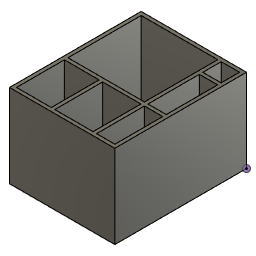
Animation v5 (Autodesk Fusion 360 archive; units mm, degrees)
design "Crate_Mid_Term"
Autodesk Fusion 360 part; units mm, degrees
note: some values were not read from the file. Set by a fixed rule: which face or edge a step refers to.
sketch "Sketch1" plane through (0, 0, 0) normal (1, 0, 0) x (0, 0, -1)
sketch "Sketch2" plane through (0, 0, 0) normal (0, 1, 0) x (1, 0, 0)
  line L0 (0, 0) -> (-24, 0)
  line L1 (-24, 0) -> (-24, -30)
  line L2 (-24, -30) -> (0, -30)
  line L3 (0, -30) -> (0, 0)
  constraint horizontal L0
  constraint vertical L1
  constraint horizontal L2
  constraint vertical L3
  constraint coincident L0.start L3.end
extrude "Extrude1" add sketch "Sketch2" along normal blind 19
sketch "Sketch3" plane through (0, 19, 0) normal (0, 1, 0) x (-1, 0, 0)
  line L0 (0, 30) -> (0, 0)
  line L1 (0, 0) -> (24, 0)
  line L2 (24, 0) -> (24, 30)
  line L3 (24, 30) -> (0, 30)
  line L4 (0.8, 0.8) -> (23.2, 0.8)
  line L5 (23.2, 0.8) -> (23.2, 29.2)
  line L6 (23.2, 29.2) -> (0.8, 29.2)
  line L7 (0.8, 29.2) -> (0.8, 0.8)
  dimension "d3" = -0.8
extrude "Extrude2" cut sketch "Sketch3" against normal blind 18.04 contours L4 L5 L6 L7
sketch "Sketch4" plane through (0, 0.96, 0) normal (0, 1, 0) x (-1, 0, 0)
  line L0 (0.8, 29.2) -> (0.8, 0.8)
  line L1 (0.8, 0.8) -> (23.2, 0.8)
  line L2 (23.2, 0.8) -> (23.2, 29.2)
  line L3 (23.2, 29.2) -> (0.8, 29.2)
  line L4 (4.9651, 0.8) -> (5.7651, 0.8)
  line L5 (5.7651, 0.8) -> (5.7651, 29.2)
  line L6 (5.7651, 29.2) -> (4.9651, 29.2)
  line L7 (4.9651, 29.2) -> (4.9651, 0.8)
  dimension "d6" = 0.8
  constraint horizontal L4
  constraint vertical L5
  constraint horizontal L6
  constraint vertical L7
  constraint coincident L3 L5.end
  constraint coincident L1 L4.start
  measures "d6" distance of L4.start L4.end
extrude "Extrude3" add sketch "Sketch4" along normal blind 18.04 contours L1 L3 L4 L5 L6 L7
sketch "Sketch5" plane through (0, 0.96, 0) normal (0, 1, 0) x (-1, 0, 0)
  line L0 (4.9651, 0.8) -> (4.9651, 29.2)
  line L1 (4.9651, 29.2) -> (0.8, 29.2)
  line L2 (0.8, 29.2) -> (0.8, 0.8)
  line L3 (0.8, 0.8) -> (4.9651, 0.8)
  line L4 (4.9651, 4.9845) -> (0.8, 4.9845)
  line L5 (0.8, 4.9845) -> (0.8, 5.7845)
  line L6 (0.8, 5.7845) -> (4.9651, 5.7845)
  line L7 (4.9651, 5.7845) -> (4.9651, 4.9845)
  dimension "d9" = 0.8
  constraint horizontal L4
  constraint vertical L5
  constraint horizontal L6
  constraint vertical L7
  constraint coincident L0 L4.start
  measures "d9" distance of L4.start L6.end
extrude "Extrude4" add sketch "Sketch5" along normal blind 18.04 contours L0 L2 L4 L5 L6 L7
sketch "Sketch6" plane through (0, 0.96, 0) normal (0, 1, 0) x (-1, 0, 0)
  line L0 (0.8, 5.7845) -> (4.9651, 5.7845)
  line L1 (4.9651, 5.7845) -> (4.9651, 29.2)
  line L2 (4.9651, 29.2) -> (0.8, 29.2)
  line L3 (0.8, 29.2) -> (0.8, 5.7845)
  line L4 (4.9651, 17.4923) -> (0.8, 17.4923)
  line L5 (0.8, 17.4923) -> (0.8, 18.2923)
  line L6 (0.8, 18.2923) -> (4.9651, 18.2923)
  line L7 (4.9651, 18.2923) -> (4.9651, 17.4923)
  dimension "d12" = 0.8
  constraint horizontal L4
  constraint vertical L5
  constraint horizontal L6
  constraint vertical L7
  constraint midpoint L1 L4.start
  measures "d12" distance of L4.start L6.end
extrude "Extrude5" add sketch "Sketch6" along normal blind 18.04 contours L1 L3 L4 L5 L6 L7
sketch "Sketch7" plane through (0, 0.96, 0) normal (0, 1, 0) x (-1, 0, 0)
  line L0 (5.7651, 29.2) -> (5.7651, 0.8)
  line L1 (5.7651, 0.8) -> (23.2, 0.8)
  line L2 (23.2, 0.8) -> (23.2, 29.2)
  line L3 (23.2, 29.2) -> (5.7651, 29.2)
  line L4 (5.7651, 17.4851) -> (23.2, 17.4851)
  line L5 (23.2, 17.4851) -> (23.2, 18.2851)
  line L6 (23.2, 18.2851) -> (5.7651, 18.2851)
  line L7 (5.7651, 18.2851) -> (5.7651, 17.4851)
  dimension "d15" = 0.8
  constraint horizontal L4
  constraint vertical L5
  constraint horizontal L6
  constraint vertical L7
  constraint coincident L0 L4.start
  measures "d15" distance of L4.start L6.end
extrude "Extrude6" add sketch "Sketch7" along normal blind 18.04 contours L0 L2 L4 L5 L6 L7
delete_face "DeleteFace1" 1 faces at (-17.3884, 6.9733, 18.2851)
sketch "Sketch8" plane through (0, 19, 0) normal (0, 1, 0) x (-1, 0, 0)
  line L0 (4.9651, 18.2923) -> (0.8, 18.2923)
  line L1 (0.8, 18.2923) -> (0.8, 29.2)
  line L2 (0.8, 29.2) -> (4.9651, 29.2)
  line L3 (4.9651, 29.2) -> (4.9651, 18.2923)
  line L4 (4.9651, 4.9845) -> (4.9651, 0.8)
  line L5 (4.9651, 0.8) -> (0.8, 0.8)
  line L6 (0.8, 0.8) -> (0.8, 4.9845)
  line L7 (0.8, 4.9845) -> (4.9651, 4.9845)
  line L8 (4.9651, 17.4923) -> (4.9651, 5.7845)
  line L9 (4.9651, 5.7845) -> (0.8, 5.7845)
  line L10 (0.8, 5.7845) -> (0.8, 17.4923)
  line L11 (0.8, 17.4923) -> (4.9651, 17.4923)
  line L12 (0, 0) -> (24, 0)
  line L13 (24, 0) -> (24, 30)
  line L14 (24, 30) -> (0, 30)
  line L15 (0, 30) -> (0, 0)
  line L16 (23.2, 17.4851) -> (23.2, 0.8)
  line L17 (23.2, 0.8) -> (5.7651, 0.8)
  line L18 (5.7651, 0.8) -> (5.7651, 17.4851)
  line L19 (5.7651, 17.4851) -> (23.2, 17.4851)
  line L20 (5.7651, 18.2923) -> (23.2, 18.2923)
  line L21 (23.2, 18.2923) -> (23.2, 29.2003)
  line L22 (23.2, 29.2003) -> (5.7651, 29.2003)
  line L23 (5.7651, 29.2003) -> (5.7651, 18.2923)
  dimension "d18" = 10.908
  constraint horizontal L20
  constraint vertical L21
  constraint horizontal L22
  constraint vertical L23
  measures "d18" distance of L20.start L22.end
extrude "Extrude7" cut sketch "Sketch8" against normal blind 18.04 contours L20 L21 L22 L23
sketch "Sketch9" plane through (0, 0.96, 0) normal (0, 1, 0) x (-1, 0, 0)
  line L0 (5.7651, 29.2003) -> (5.7651, 18.2923)
  line L1 (5.7651, 18.2923) -> (23.2, 18.2923)
  line L2 (23.2, 18.2923) -> (23.2, 29.2003)
  line L3 (23.2, 29.2003) -> (5.7651, 29.2003)
  line L4 (14.4825, 18.2923) -> (15.2825, 18.2923)
  line L5 (15.2825, 18.2923) -> (15.2825, 29.2003)
  line L6 (15.2825, 29.2003) -> (14.4825, 29.2003)
  line L7 (14.4825, 29.2003) -> (14.4825, 18.2923)
  dimension "d21" = 0.8
  constraint horizontal L4
  constraint vertical L5
  constraint horizontal L6
  constraint vertical L7
  constraint midpoint L1 L4.start
  measures "d21" distance of L4.start L4.end
extrude "Extrude8" add sketch "Sketch9" along normal blind 18.04 contours L1 L3 L4 L5 L6 L7

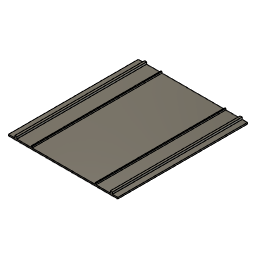
design "Floor"
Autodesk Fusion 360 part; units mm, degrees
sketch "Sketch1" plane through (0, 0, 0) normal (0, 1, 0) x (1, 0, 0)
  line L0 (0, 0) -> (-140, 0)
  line L1 (-140, 0) -> (-140, 140)
  line L2 (-140, 140) -> (0, 140)
  line L3 (0, 140) -> (0, 0)
  dimension "d1" = 140
  dimension "d2" = 140
  constraint horizontal L0
  constraint vertical L1
  constraint horizontal L2
  constraint vertical L3
  constraint coincident L0.start L3.end
  measures "d1" distance of L0.start L0.end
  measures "d2" distance of L0.start L2.end
extrude "Extrude1" add sketch "Sketch1" along normal blind 2 makes body 1
sketch "Sketch2" plane through (0, 2, 0) normal (0, 1, 0) x (-1, 0, 0)
  line L0 (0, -140) -> (140, -140)
  line L1 (140, -140) -> (140, 0)
  line L2 (140, 0) -> (0, 0)
  line L3 (0, 0) -> (0, -140)
  line L4 (70, -140) -> (23, -140)
  line L5 (117, -140) -> (116, -140)
  line L6 (117, -140) -> (117.75, -140)
  line L7 (117.75, -140) -> (116.25, -140)
  line L8 (117.75, -140) -> (116.25, -140)
  line L9 (116.25, -140) -> (116.25, 0)
  line L10 (116.25, 0) -> (117.75, 0)
  line L11 (117.75, 0) -> (117.75, -140)
  dimension "d5" = 47
  dimension "d6" = 47
  dimension "d7" = 0.75
  dimension "d8" = 1.5
  constraint midpoint L0 L4.start
  constraint parallel L0 L4
  constraint parallel L0 L6
  constraint horizontal L7
  constraint horizontal L8
  constraint vertical L9
  constraint horizontal L10
  constraint vertical L11
  constraint coincident L2 L9.end
  measures "d5" distance of L4.start L5.start
  measures "d6" distance of L4.start L4.end
  measures "d7" distance of L5.start L6.end
  measures "d8" distance of L6.end L7.end
extrude "Extrude2" add sketch "Sketch2" along normal blind 2 contours L0 L2 L5 L6 L7 L8 L9 L10 L11 bodies 1
sketch "Sketch3" plane through (0, 2, 0) normal (0, 1, 0) x (-1, 0, 0)
  line L0 (116.25, -140) -> (116.25, 0)
  line L1 (116.25, 0) -> (0, 0)
  line L2 (0, 0) -> (0, -140)
  line L3 (0, -140) -> (116.25, -140)
  line L4 (0, -140) -> (22.25, -140)
  line L5 (22.25, -140) -> (20.75, -140)
  line L6 (20.75, -140) -> (20.75, 0)
  line L7 (20.75, 0) -> (22.25, 0)
  line L8 (22.25, 0) -> (22.25, -140)
  dimension "d11" = 22.25
  dimension "d12" = 1.5
  constraint coincident L2.end L3.start
  constraint perpendicular L2 L4
  constraint horizontal L5
  constraint vertical L6
  constraint horizontal L7
  constraint vertical L8
  measures "d11" distance of L2.end L4.end
  measures "d12" distance of L4.end L5.end
extrude "Extrude3" add sketch "Sketch3" along normal blind 2 contours L1 L3 L4 L5 L6 L7 L8 bodies 1
sketch "Sketch4" plane through (0, 2, 0) normal (0, 1, 0) x (-1, 0, 0)
extrude "Extrude4" add 1 faces at (0, 0.6667, -93.3333) along direction (1, 0, 0) blind 10 on bodies 1 bodies 1
extrude "Extrude5" add 1 faces at (-140, 0.6667, -46.6667) along direction (-1, 0, 0) blind 10 on bodies 1 bodies 1
sketch "Sketch5" plane through (0, 2, 0) normal (0, 1, 0) x (-1, 0, 0)
  line L0 (20.75, -140) -> (20.75, 0)
  line L1 (20.75, 0) -> (-10, 0)
  line L2 (-10, 0) -> (-10, -140)
  line L3 (-10, -140) -> (20.75, -140)
  line L4 (0.75, -140) -> (-2.25, -140)
  line L5 (-2.25, -140) -> (-2.25, 0)
  line L6 (-2.25, 0) -> (0.75, 0)
  line L7 (0.75, 0) -> (0.75, -140)
  dimension "d19" = 20
  dimension "d20" = 3
  dimension "d21" = 140
  constraint horizontal L4
  constraint vertical L5
  constraint horizontal L6
  constraint vertical L7
  measures "d19" distance of L0.start L4.start
  measures "d20" distance of L4.start L4.end
  measures "d21" distance of L4.start L6.end
extrude "Extrude6" add sketch "Sketch5" along normal blind 3 contours L1 L3 L4 L5 L6 L7 bodies 1
sketch "Sketch6" plane through (0, 2, 0) normal (0, 1, 0) x (-1, 0, 0)
  line L0 (117.75, 0) -> (117.75, -140)
  line L1 (117.75, -140) -> (150, -140)
  line L2 (150, -140) -> (150, 0)
  line L3 (150, 0) -> (117.75, 0)
  line L4 (137.75, -140) -> (140.75, -140)
  line L5 (140.75, -140) -> (140.75, 0)
  line L6 (140.75, 0) -> (137.75, 0)
  line L7 (137.75, 0) -> (137.75, -140)
  dimension "d24" = 20
  dimension "d25" = 3
  dimension "d26" = 140
  constraint horizontal L4
  constraint vertical L5
  constraint horizontal L6
  constraint vertical L7
  measures "d24" distance of L0.end L4.start
  measures "d25" distance of L4.start L4.end
  measures "d26" distance of L4.start L6.end
extrude "Extrude7" add sketch "Sketch6" along normal blind 3 contours L1 L3 L4 L5 L6 L7 bodies 1
sketch "Sketch7" plane through (0, 5, 0) normal (0, 1, 0) x (-1, 0, 0)
sketch "Sketch8" plane through (0, 2, 0) normal (0, 1, 0) x (-1, 0, 0)
sketch "Sketch9" plane through (0, 5, 0) normal (0, 1, 0) x (-1, 0, 0)
sketch "Sketch10" plane through (0, 5, 0) normal (0, 1, 0) x (-1, 0, 0)
sketch "Sketch11" plane through (0, 2, 0) normal (0, 1, 0) x (-1, 0, 0)
  line L0 (22.25, -140) -> (116.25, -140)
  line L1 (116.25, -140) -> (116.25, 0)
  line L2 (116.25, 0) -> (22.25, 0)
  line L3 (23.25, 0) -> (21.75, 0)
  line L4 (21.75, 0) -> (21.75, -140)
  line L5 (21.75, -140) -> (23.25, -140)
  line L6 (23.25, -140) -> (23.25, 0)
  dimension "d29" = 1
  dimension "d30" = 1.5
  constraint horizontal L3
  constraint vertical L4
  constraint horizontal L5
  constraint vertical L6
  measures "d29" distance of L2.end L3.start
  measures "d30" distance of L3.start L3.end
extrude "Extrude8" cut 1 faces at (-21.75, 4, -93.3333) along direction (0, -1, 0) blind 2 on bodies 1 bodies 1
extrude "Extrude9" add sketch "Sketch11" along normal blind 2 contours L0 L2 L3 L4 L5 L6 bodies 1
extrude "Extrude10" cut 1 faces at (-116.75, 4, -93.3333) along direction (0, -1, 0) blind 2 on bodies 1 bodies 1
sketch "Sketch12" plane through (0, 2, 0) normal (0, 1, 0) x (-1, 0, 0)
  line L0 (23.25, 0) -> (23.25, -140)
  line L1 (23.25, -140) -> (137.75, -140)
  line L2 (137.75, -140) -> (137.75, 0)
  line L3 (137.75, 0) -> (23.25, 0)
  line L4 (23.25, -140) -> (115.25, -140)
  line L5 (115.25, -140) -> (116.75, -140)
  line L6 (116.75, -140) -> (116.75, 0)
  line L7 (116.75, 0) -> (115.25, 0)
  line L8 (115.25, 0) -> (115.25, -140)
  dimension "d37" = 92
  dimension "d38" = 1.5
  constraint coincident L0.end L1.start
  constraint perpendicular L0 L4
  constraint horizontal L5
  constraint vertical L6
  constraint horizontal L7
  constraint vertical L8
  measures "d37" distance of L0.end L4.end
  measures "d38" distance of L4.end L5.end
extrude "Extrude11" add sketch "Sketch12" along normal blind 2 contours L1 L3 L5 L6 L7 L8 bodies 1
sketch "Sketch13" plane through (0, 2, 0) normal (0, 1, 0) x (-1, 0, 0)
copy_body "Body->Comp1" bodies 1 removing the originals makes body 2 in component "Component"
extrude "Extrude1'" add 1 faces at (-92.5833, 0.6667, 0) along direction (0, 0, 1) blind 50 on bodies 2 bodies 2 in component "Component"
component "Component" placed x (1, 0, 0) y (0, 1, 0) z (0, 0, 1) at (0, 0, 0)

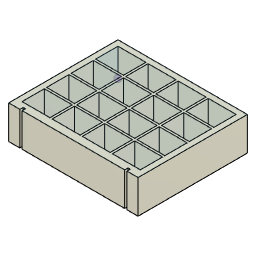
design "Cabinet"
Autodesk Fusion 360 part; units mm, degrees
sketch "Sketch1" plane through (0, 0, 0) normal (0, 1, 0) x (1, 0, 0)
sketch "Sketch2" plane through (0, 0, 0) normal (0, 1, 0) x (1, 0, 0)
sketch "Sketch3" plane through (0, 0, 0) normal (0, 1, 0) x (1, 0, 0)
  line L0 (-10, 10) -> (100, 10)
  line L1 (100, 10) -> (100, -80)
  line L2 (100, -80) -> (-10, -80)
  line L3 (-10, -80) -> (-10, 10)
  constraint horizontal L0
  constraint vertical L1
  constraint horizontal L2
  constraint vertical L3
sketch "Sketch4" plane through (0, 0, 0) normal (0, 1, 0) x (1, 0, 0)
sketch "Sketch5" plane through (0, 0, 0) normal (0, 1, 0) x (1, 0, 0)
  line L0 (0, 0) -> (116, 0)
  line L1 (116, 0) -> (116, -98)
  line L2 (116, -98) -> (0, -98)
  line L3 (0, -98) -> (0, 0)
  dimension "d4" = 116
  dimension "d5" = 98
  constraint horizontal L0
  constraint vertical L1
  constraint horizontal L2
  constraint vertical L3
  constraint coincident L0.start L3.end
  measures "d4" distance of L0.start L0.end
  measures "d5" distance of L0.start L2.end
extrude "Extrude2" add sketch "Sketch5" along normal blind 30
shell "Shell2" thickness 5 removed faces 1 at (38.6667, 30, 32.6667)
delete_face "DeleteFace2" 1 faces at (40.3333, 5, 34.3333)
sketch "Sketch6" plane through (0, 0, 0) normal (0, 1, 0) x (1, 0, 0)
  line L0 (5, -5) -> (32, -5)
  line L1 (32, -5) -> (32, -27)
  line L2 (32, -27) -> (5, -27)
  line L3 (5, -27) -> (5, -5)
  dimension "d9" = 27
  dimension "d10" = 22
  constraint horizontal L0
  constraint vertical L1
  constraint horizontal L2
  constraint vertical L3
  measures "d9" distance of L0.start L0.end
  measures "d10" distance of L0.start L2.end
extrude "Extrude3" add sketch "Sketch6" along normal blind 30
sketch "Sketch7" plane through (0, 30, 0) normal (0, 1, 0) x (-1, 0, 0)
  line L0 (-116, 98) -> (-116, 0)
  line L1 (-116, 0) -> (0, 0)
  line L2 (0, 0) -> (0, 98)
  line L3 (0, 98) -> (-116, 98)
  line L4 (-111, 93) -> (-5, 93)
  line L5 (-5, 93) -> (-5, 27)
  line L6 (-5, 27) -> (-32, 27)
  line L7 (-32, 27) -> (-32, 5)
  line L8 (-32, 5) -> (-111, 5)
  line L9 (-111, 5) -> (-111, 93)
  line L10 (-5, 5) -> (-30, 5)
  line L11 (-30, 5) -> (-30, 25)
  line L12 (-30, 25) -> (-5, 25)
  line L13 (-5, 25) -> (-5, 5)
  constraint horizontal L10
  constraint vertical L11
  constraint horizontal L12
  constraint vertical L13
extrude "Extrude4" cut sketch "Sketch7" against normal blind 30 contours L10 L11 L12 L13
sketch "Sketch8" plane through (0, 0, 0) normal (0, 1, 0) x (1, 0, 0)
  line L0 (32, -5) -> (59, -5)
  line L1 (59, -5) -> (59, -27)
  line L2 (59, -27) -> (32, -27)
  line L3 (32, -27) -> (32, -5)
  dimension "d15" = 27
  dimension "d16" = 22
  constraint horizontal L0
  constraint vertical L1
  constraint horizontal L2
  constraint vertical L3
  measures "d15" distance of L0.start L0.end
  measures "d16" distance of L0.start L2.end
extrude "Extrude5" add sketch "Sketch8" along normal blind 30
sketch "Sketch9" plane through (0, 30, 0) normal (0, 1, 0) x (-1, 0, 0)
  line L0 (-30, 5) -> (-30, 25)
  line L1 (-30, 25) -> (-5, 25)
  line L2 (-5, 25) -> (-5, 5)
  line L3 (-5, 5) -> (-30, 5)
  line L4 (-116, 98) -> (-116, 0)
  line L5 (-116, 0) -> (0, 0)
  line L6 (0, 0) -> (0, 98)
  line L7 (0, 98) -> (-116, 98)
  line L8 (-111, 93) -> (-5, 93)
  line L9 (-5, 93) -> (-5, 27)
  line L10 (-5, 27) -> (-59, 27)
  line L11 (-59, 27) -> (-59, 5)
  line L12 (-59, 5) -> (-111, 5)
  line L13 (-111, 5) -> (-111, 93)
  line L14 (-32, 5) -> (-57, 5)
  line L15 (-57, 5) -> (-57, 25)
  line L16 (-57, 25) -> (-32, 25)
  line L17 (-32, 25) -> (-32, 5)
  constraint horizontal L14
  constraint vertical L15
  constraint horizontal L16
  constraint vertical L17
extrude "Extrude6" cut sketch "Sketch9" against normal blind 30 contours L14 L15 L16 L17
sketch "Sketch10" plane through (0, 0, 0) normal (0, 1, 0) x (1, 0, 0)
  line L0 (59, -5) -> (86, -5)
  line L1 (86, -5) -> (86, -27)
  line L2 (86, -27) -> (59, -27)
  line L3 (59, -27) -> (59, -5)
  dimension "d21" = 27
  dimension "d22" = 22
  constraint horizontal L0
  constraint vertical L1
  constraint horizontal L2
  constraint vertical L3
  measures "d21" distance of L0.start L0.end
  measures "d22" distance of L0.start L2.end
extrude "Extrude7" add sketch "Sketch10" along normal blind 30
sketch "Sketch11" plane through (0, 30, 0) normal (0, 1, 0) x (-1, 0, 0)
  line L0 (-57, 5) -> (-57, 25)
  line L1 (-57, 25) -> (-32, 25)
  line L2 (-32, 25) -> (-32, 5)
  line L3 (-32, 5) -> (-57, 5)
  line L4 (-30, 5) -> (-30, 25)
  line L5 (-30, 25) -> (-5, 25)
  line L6 (-5, 25) -> (-5, 5)
  line L7 (-5, 5) -> (-30, 5)
  line L8 (-116, 98) -> (-116, 0)
  line L9 (-116, 0) -> (0, 0)
  line L10 (0, 0) -> (0, 98)
  line L11 (0, 98) -> (-116, 98)
  line L12 (-111, 93) -> (-5, 93)
  line L13 (-5, 93) -> (-5, 27)
  line L14 (-5, 27) -> (-86, 27)
  line L15 (-86, 27) -> (-86, 5)
  line L16 (-86, 5) -> (-111, 5)
  line L17 (-111, 5) -> (-111, 93)
  line L18 (-59, 5) -> (-84, 5)
  line L19 (-84, 5) -> (-84, 25)
  line L20 (-84, 25) -> (-59, 25)
  line L21 (-59, 25) -> (-59, 5)
  constraint horizontal L18
  constraint vertical L19
  constraint horizontal L20
  constraint vertical L21
extrude "Extrude8" cut sketch "Sketch11" against normal blind 30 contours L18 L19 L20 L21
sketch "Sketch12" plane through (0, 0, 0) normal (0, 1, 0) x (1, 0, 0)
  line L0 (86, -27) -> (111, -27)
  line L1 (111, -27) -> (111, -5)
  line L2 (111, -5) -> (86, -5)
  line L3 (86, -5) -> (86, -27)
  constraint horizontal L0
  constraint vertical L1
  constraint horizontal L2
  constraint vertical L3
extrude "Extrude9" add sketch "Sketch12" along normal blind 30
sketch "Sketch13" plane through (0, 30, 0) normal (0, 1, 0) x (-1, 0, 0)
  line L0 (-84, 5) -> (-84, 25)
  line L1 (-84, 25) -> (-59, 25)
  line L2 (-59, 25) -> (-59, 5)
  line L3 (-59, 5) -> (-84, 5)
  line L4 (-57, 5) -> (-57, 25)
  line L5 (-57, 25) -> (-32, 25)
  line L6 (-32, 25) -> (-32, 5)
  line L7 (-32, 5) -> (-57, 5)
  line L8 (-30, 5) -> (-30, 25)
  line L9 (-30, 25) -> (-5, 25)
  line L10 (-5, 25) -> (-5, 5)
  line L11 (-5, 5) -> (-30, 5)
  line L12 (-116, 98) -> (-116, 0)
  line L13 (-116, 0) -> (0, 0)
  line L14 (0, 0) -> (0, 98)
  line L15 (0, 98) -> (-116, 98)
  line L16 (-111, 93) -> (-5, 93)
  line L17 (-5, 93) -> (-5, 27)
  line L18 (-5, 27) -> (-111, 27)
  line L19 (-111, 27) -> (-111, 93)
  line L20 (-86, 25) -> (-111, 25)
  line L21 (-111, 25) -> (-111, 5)
  line L22 (-111, 5) -> (-86, 5)
  line L23 (-86, 5) -> (-86, 25)
  constraint horizontal L20
  constraint vertical L21
  constraint horizontal L22
  constraint vertical L23
extrude "Extrude10" cut sketch "Sketch13" against normal blind 30 contours L20 L21 L22 L23
sketch "Sketch14" plane through (0, 0, 0) normal (0, 1, 0) x (1, 0, 0)
  line L0 (5, -27) -> (32, -27)
  line L1 (32, -27) -> (32, -49)
  line L2 (32, -49) -> (5, -49)
  line L3 (5, -49) -> (5, -27)
  constraint horizontal L0
  constraint vertical L1
  constraint horizontal L2
  constraint vertical L3
extrude "Extrude11" add sketch "Sketch14" along normal blind 30
sketch "Sketch15" plane through (0, 30, 0) normal (0, 1, 0) x (-1, 0, 0)
  line L0 (-111, 25) -> (-86, 25)
  line L1 (-86, 25) -> (-86, 5)
  line L2 (-86, 5) -> (-111, 5)
  line L3 (-111, 5) -> (-111, 25)
  line L4 (-84, 5) -> (-84, 25)
  line L5 (-84, 25) -> (-59, 25)
  line L6 (-59, 25) -> (-59, 5)
  line L7 (-59, 5) -> (-84, 5)
  line L8 (-57, 5) -> (-57, 25)
  line L9 (-57, 25) -> (-32, 25)
  line L10 (-32, 25) -> (-32, 5)
  line L11 (-32, 5) -> (-57, 5)
  line L12 (-30, 5) -> (-30, 25)
  line L13 (-30, 25) -> (-5, 25)
  line L14 (-5, 25) -> (-5, 5)
  line L15 (-5, 5) -> (-30, 5)
  line L16 (-116, 98) -> (-116, 0)
  line L17 (-116, 0) -> (0, 0)
  line L18 (0, 0) -> (0, 98)
  line L19 (0, 98) -> (-116, 98)
  line L20 (-111, 93) -> (-5, 93)
  line L21 (-5, 93) -> (-5, 49)
  line L22 (-5, 49) -> (-32, 49)
  line L23 (-32, 49) -> (-32, 27)
  line L24 (-32, 27) -> (-111, 27)
  line L25 (-111, 27) -> (-111, 93)
  line L26 (-5, 27) -> (-30, 27)
  line L27 (-30, 27) -> (-30, 47)
  line L28 (-30, 47) -> (-5, 47)
  line L29 (-5, 47) -> (-5, 27)
  constraint horizontal L26
  constraint vertical L27
  constraint horizontal L28
  constraint vertical L29
extrude "Extrude12" cut sketch "Sketch15" against normal blind 30 contours L26 L27 L28 L29
sketch "Sketch16" plane through (5, 0, 0) normal (1, 0, 0) x (0, 0, -1)
  line L0 (-5, 30) -> (-25, 30)
  line L1 (-25, 30) -> (-25, 0)
  line L2 (-25, 0) -> (-5, 0)
  line L3 (-5, 0) -> (-5, 30)
sketch "Sketch17" plane through (0, 0, 0) normal (0, 1, 0) x (1, 0, 0)
  line L0 (32, -49) -> (59, -49)
  line L1 (59, -49) -> (59, -27)
  line L2 (59, -27) -> (32, -27)
  line L3 (32, -27) -> (32, -49)
  constraint horizontal L0
  constraint vertical L1
  constraint horizontal L2
  constraint vertical L3
extrude "Extrude13" add sketch "Sketch17" along normal blind 30
sketch "Sketch18" plane through (0, 30, 0) normal (0, 1, 0) x (-1, 0, 0)
  line L0 (-30, 27) -> (-30, 47)
  line L1 (-30, 47) -> (-5, 47)
  line L2 (-5, 47) -> (-5, 27)
  line L3 (-5, 27) -> (-30, 27)
  line L4 (-111, 25) -> (-86, 25)
  line L5 (-86, 25) -> (-86, 5)
  line L6 (-86, 5) -> (-111, 5)
  line L7 (-111, 5) -> (-111, 25)
  line L8 (-84, 5) -> (-84, 25)
  line L9 (-84, 25) -> (-59, 25)
  line L10 (-59, 25) -> (-59, 5)
  line L11 (-59, 5) -> (-84, 5)
  line L12 (-57, 5) -> (-57, 25)
  line L13 (-57, 25) -> (-32, 25)
  line L14 (-32, 25) -> (-32, 5)
  line L15 (-32, 5) -> (-57, 5)
  line L16 (-30, 5) -> (-30, 25)
  line L17 (-30, 25) -> (-5, 25)
  line L18 (-5, 25) -> (-5, 5)
  line L19 (-5, 5) -> (-30, 5)
  line L20 (-116, 98) -> (-116, 0)
  line L21 (-116, 0) -> (0, 0)
  line L22 (0, 0) -> (0, 98)
  line L23 (0, 98) -> (-116, 98)
  line L24 (-111, 93) -> (-5, 93)
  line L25 (-5, 93) -> (-5, 49)
  line L26 (-5, 49) -> (-59, 49)
  line L27 (-59, 49) -> (-59, 27)
  line L28 (-59, 27) -> (-111, 27)
  line L29 (-111, 27) -> (-111, 93)
  line L30 (-32, 27) -> (-57, 27)
  line L31 (-57, 27) -> (-57, 47)
  line L32 (-57, 47) -> (-32, 47)
  line L33 (-32, 47) -> (-32, 27)
  constraint horizontal L30
  constraint vertical L31
  constraint horizontal L32
  constraint vertical L33
extrude "Extrude14" cut sketch "Sketch18" against normal blind 30 contours L30 L31 L32 L33
sketch "Sketch19" plane through (0, 0, 0) normal (0, 1, 0) x (1, 0, 0)
  line L0 (59, -49) -> (86, -49)
  line L1 (86, -49) -> (86, -27)
  line L2 (86, -27) -> (59, -27)
  line L3 (59, -27) -> (59, -49)
  constraint horizontal L0
  constraint vertical L1
  constraint horizontal L2
  constraint vertical L3
extrude "Extrude15" add sketch "Sketch19" along normal blind 30
sketch "Sketch20" plane through (0, 0, 0) normal (0, 1, 0) x (1, 0, 0)
  line L0 (86, -27) -> (111, -27)
  line L1 (111, -27) -> (111, -49)
  line L2 (111, -49) -> (86, -49)
  line L3 (86, -49) -> (86, -27)
  constraint horizontal L0
  constraint vertical L1
  constraint horizontal L2
  constraint vertical L3
extrude "Extrude16" add sketch "Sketch20" along normal blind 30
sketch "Sketch21" plane through (0, 30, 0) normal (0, 1, 0) x (-1, 0, 0)
  line L0 (-57, 27) -> (-57, 47)
  line L1 (-57, 47) -> (-32, 47)
  line L2 (-32, 47) -> (-32, 27)
  line L3 (-32, 27) -> (-57, 27)
  line L4 (-30, 27) -> (-30, 47)
  line L5 (-30, 47) -> (-5, 47)
  line L6 (-5, 47) -> (-5, 27)
  line L7 (-5, 27) -> (-30, 27)
  line L8 (-111, 25) -> (-86, 25)
  line L9 (-86, 25) -> (-86, 5)
  line L10 (-86, 5) -> (-111, 5)
  line L11 (-111, 5) -> (-111, 25)
  line L12 (-84, 5) -> (-84, 25)
  line L13 (-84, 25) -> (-59, 25)
  line L14 (-59, 25) -> (-59, 5)
  line L15 (-59, 5) -> (-84, 5)
  line L16 (-57, 5) -> (-57, 25)
  line L17 (-57, 25) -> (-32, 25)
  line L18 (-32, 25) -> (-32, 5)
  line L19 (-32, 5) -> (-57, 5)
  line L20 (-30, 5) -> (-30, 25)
  line L21 (-30, 25) -> (-5, 25)
  line L22 (-5, 25) -> (-5, 5)
  line L23 (-5, 5) -> (-30, 5)
  line L24 (-116, 98) -> (-116, 0)
  line L25 (-116, 0) -> (0, 0)
  line L26 (0, 0) -> (0, 98)
  line L27 (0, 98) -> (-116, 98)
  line L28 (-111, 93) -> (-5, 93)
  line L29 (-5, 93) -> (-5, 49)
  line L30 (-5, 49) -> (-111, 49)
  line L31 (-111, 49) -> (-111, 93)
  line L32 (-59, 27) -> (-84, 27)
  line L33 (-84, 27) -> (-84, 47)
  line L34 (-84, 47) -> (-59, 47)
  line L35 (-59, 47) -> (-59, 27)
  constraint horizontal L32
  constraint vertical L33
  constraint horizontal L34
  constraint vertical L35
extrude "Extrude17" cut sketch "Sketch21" against normal blind 30 contours L32 L33 L34 L35
sketch "Sketch22" plane through (0, 30, 0) normal (0, 1, 0) x (-1, 0, 0)
  line L0 (-84, 27) -> (-84, 47)
  line L1 (-84, 47) -> (-59, 47)
  line L2 (-59, 47) -> (-59, 27)
  line L3 (-59, 27) -> (-84, 27)
  line L4 (-57, 27) -> (-57, 47)
  line L5 (-57, 47) -> (-32, 47)
  line L6 (-32, 47) -> (-32, 27)
  line L7 (-32, 27) -> (-57, 27)
  line L8 (-30, 27) -> (-30, 47)
  line L9 (-30, 47) -> (-5, 47)
  line L10 (-5, 47) -> (-5, 27)
  line L11 (-5, 27) -> (-30, 27)
  line L12 (-111, 25) -> (-86, 25)
  line L13 (-86, 25) -> (-86, 5)
  line L14 (-86, 5) -> (-111, 5)
  line L15 (-111, 5) -> (-111, 25)
  line L16 (-84, 5) -> (-84, 25)
  line L17 (-84, 25) -> (-59, 25)
  line L18 (-59, 25) -> (-59, 5)
  line L19 (-59, 5) -> (-84, 5)
  line L20 (-57, 5) -> (-57, 25)
  line L21 (-57, 25) -> (-32, 25)
  line L22 (-32, 25) -> (-32, 5)
  line L23 (-32, 5) -> (-57, 5)
  line L24 (-30, 5) -> (-30, 25)
  line L25 (-30, 25) -> (-5, 25)
  line L26 (-5, 25) -> (-5, 5)
  line L27 (-5, 5) -> (-30, 5)
  line L28 (-116, 98) -> (-116, 0)
  line L29 (-116, 0) -> (0, 0)
  line L30 (0, 0) -> (0, 98)
  line L31 (0, 98) -> (-116, 98)
  line L32 (-111, 93) -> (-5, 93)
  line L33 (-5, 93) -> (-5, 49)
  line L34 (-5, 49) -> (-111, 49)
  line L35 (-111, 49) -> (-111, 93)
  line L36 (-86, 27) -> (-111, 27)
  line L37 (-111, 27) -> (-111, 47)
  line L38 (-111, 47) -> (-86, 47)
  line L39 (-86, 47) -> (-86, 27)
  constraint horizontal L36
  constraint vertical L37
  constraint horizontal L38
  constraint vertical L39
extrude "Extrude18" cut sketch "Sketch22" against normal blind 30 contours L36 L37 L38 L39
sketch "Sketch23" plane through (0, 0, 0) normal (0, 1, 0) x (1, 0, 0)
  line L0 (5, -49) -> (111, -49)
  line L1 (111, -49) -> (111, -93)
  line L2 (111, -93) -> (5, -93)
  line L3 (5, -93) -> (5, -49)
  constraint horizontal L0
  constraint vertical L1
  constraint horizontal L2
  constraint vertical L3
extrude "Extrude19" add sketch "Sketch23" along normal blind 30
sketch "Sketch24" plane through (0, 30, 0) normal (0, 1, 0) x (-1, 0, 0)
  line L0 (-111, 27) -> (-111, 47)
  line L1 (-111, 47) -> (-86, 47)
  line L2 (-86, 47) -> (-86, 27)
  line L3 (-86, 27) -> (-111, 27)
  line L4 (-84, 27) -> (-84, 47)
  line L5 (-84, 47) -> (-59, 47)
  line L6 (-59, 47) -> (-59, 27)
  line L7 (-59, 27) -> (-84, 27)
  line L8 (-57, 27) -> (-57, 47)
  line L9 (-57, 47) -> (-32, 47)
  line L10 (-32, 47) -> (-32, 27)
  line L11 (-32, 27) -> (-57, 27)
  line L12 (-30, 27) -> (-30, 47)
  line L13 (-30, 47) -> (-5, 47)
  line L14 (-5, 47) -> (-5, 27)
  line L15 (-5, 27) -> (-30, 27)
  line L16 (-111, 25) -> (-86, 25)
  line L17 (-86, 25) -> (-86, 5)
  line L18 (-86, 5) -> (-111, 5)
  line L19 (-111, 5) -> (-111, 25)
  line L20 (-84, 5) -> (-84, 25)
  line L21 (-84, 25) -> (-59, 25)
  line L22 (-59, 25) -> (-59, 5)
  line L23 (-59, 5) -> (-84, 5)
  line L24 (-57, 5) -> (-57, 25)
  line L25 (-57, 25) -> (-32, 25)
  line L26 (-32, 25) -> (-32, 5)
  line L27 (-32, 5) -> (-57, 5)
  line L28 (-30, 5) -> (-30, 25)
  line L29 (-30, 25) -> (-5, 25)
  line L30 (-5, 25) -> (-5, 5)
  line L31 (-5, 5) -> (-30, 5)
  line L32 (-116, 98) -> (-116, 0)
  line L33 (-116, 0) -> (0, 0)
  line L34 (0, 0) -> (0, 98)
  line L35 (0, 98) -> (-116, 98)
  line L36 (-5, 49) -> (-30, 49)
  line L37 (-30, 49) -> (-30, 69)
  line L38 (-30, 69) -> (-5, 69)
  line L39 (-5, 69) -> (-5, 49)
  constraint horizontal L36
  constraint vertical L37
  constraint horizontal L38
  constraint vertical L39
extrude "Extrude20" cut sketch "Sketch24" against normal blind 30 contours L36 L37 L38 L39
sketch "Sketch25" plane through (0, 30, 0) normal (0, 1, 0) x (-1, 0, 0)
  line L0 (-30, 49) -> (-30, 69)
  line L1 (-30, 69) -> (-5, 69)
  line L2 (-5, 69) -> (-5, 49)
  line L3 (-5, 49) -> (-30, 49)
  line L4 (-111, 27) -> (-111, 47)
  line L5 (-111, 47) -> (-86, 47)
  line L6 (-86, 47) -> (-86, 27)
  line L7 (-86, 27) -> (-111, 27)
  line L8 (-84, 27) -> (-84, 47)
  line L9 (-84, 47) -> (-59, 47)
  line L10 (-59, 47) -> (-59, 27)
  line L11 (-59, 27) -> (-84, 27)
  line L12 (-57, 27) -> (-57, 47)
  line L13 (-57, 47) -> (-32, 47)
  line L14 (-32, 47) -> (-32, 27)
  line L15 (-32, 27) -> (-57, 27)
  line L16 (-30, 27) -> (-30, 47)
  line L17 (-30, 47) -> (-5, 47)
  line L18 (-5, 47) -> (-5, 27)
  line L19 (-5, 27) -> (-30, 27)
  line L20 (-111, 25) -> (-86, 25)
  line L21 (-86, 25) -> (-86, 5)
  line L22 (-86, 5) -> (-111, 5)
  line L23 (-111, 5) -> (-111, 25)
  line L24 (-84, 5) -> (-84, 25)
  line L25 (-84, 25) -> (-59, 25)
  line L26 (-59, 25) -> (-59, 5)
  line L27 (-59, 5) -> (-84, 5)
  line L28 (-57, 5) -> (-57, 25)
  line L29 (-57, 25) -> (-32, 25)
  line L30 (-32, 25) -> (-32, 5)
  line L31 (-32, 5) -> (-57, 5)
  line L32 (-30, 5) -> (-30, 25)
  line L33 (-30, 25) -> (-5, 25)
  line L34 (-5, 25) -> (-5, 5)
  line L35 (-5, 5) -> (-30, 5)
  line L36 (-116, 98) -> (-116, 0)
  line L37 (-116, 0) -> (0, 0)
  line L38 (0, 0) -> (0, 98)
  line L39 (0, 98) -> (-116, 98)
  line L40 (-32, 49) -> (-57, 49)
  line L41 (-57, 49) -> (-57, 69)
  line L42 (-57, 69) -> (-32, 69)
  line L43 (-32, 69) -> (-32, 49)
  constraint horizontal L40
  constraint vertical L41
  constraint horizontal L42
  constraint vertical L43
extrude "Extrude21" cut sketch "Sketch25" against normal blind 30 contours L40 L41 L42 L43
sketch "Sketch26" plane through (0, 30, 0) normal (0, 1, 0) x (-1, 0, 0)
  line L0 (-57, 49) -> (-57, 69)
  line L1 (-57, 69) -> (-32, 69)
  line L2 (-32, 69) -> (-32, 49)
  line L3 (-32, 49) -> (-57, 49)
  line L4 (-30, 49) -> (-30, 69)
  line L5 (-30, 69) -> (-5, 69)
  line L6 (-5, 69) -> (-5, 49)
  line L7 (-5, 49) -> (-30, 49)
  line L8 (-111, 27) -> (-111, 47)
  line L9 (-111, 47) -> (-86, 47)
  line L10 (-86, 47) -> (-86, 27)
  line L11 (-86, 27) -> (-111, 27)
  line L12 (-84, 27) -> (-84, 47)
  line L13 (-84, 47) -> (-59, 47)
  line L14 (-59, 47) -> (-59, 27)
  line L15 (-59, 27) -> (-84, 27)
  line L16 (-57, 27) -> (-57, 47)
  line L17 (-57, 47) -> (-32, 47)
  line L18 (-32, 47) -> (-32, 27)
  line L19 (-32, 27) -> (-57, 27)
  line L20 (-30, 27) -> (-30, 47)
  line L21 (-30, 47) -> (-5, 47)
  line L22 (-5, 47) -> (-5, 27)
  line L23 (-5, 27) -> (-30, 27)
  line L24 (-111, 25) -> (-86, 25)
  line L25 (-86, 25) -> (-86, 5)
  line L26 (-86, 5) -> (-111, 5)
  line L27 (-111, 5) -> (-111, 25)
  line L28 (-84, 5) -> (-84, 25)
  line L29 (-84, 25) -> (-59, 25)
  line L30 (-59, 25) -> (-59, 5)
  line L31 (-59, 5) -> (-84, 5)
  line L32 (-57, 5) -> (-57, 25)
  line L33 (-57, 25) -> (-32, 25)
  line L34 (-32, 25) -> (-32, 5)
  line L35 (-32, 5) -> (-57, 5)
  line L36 (-30, 5) -> (-30, 25)
  line L37 (-30, 25) -> (-5, 25)
  line L38 (-5, 25) -> (-5, 5)
  line L39 (-5, 5) -> (-30, 5)
  line L40 (-116, 98) -> (-116, 0)
  line L41 (-116, 0) -> (0, 0)
  line L42 (0, 0) -> (0, 98)
  line L43 (0, 98) -> (-116, 98)
  line L44 (-59, 49) -> (-84, 49)
  line L45 (-84, 49) -> (-84, 69)
  line L46 (-84, 69) -> (-59, 69)
  line L47 (-59, 69) -> (-59, 49)
  constraint horizontal L44
  constraint vertical L45
  constraint horizontal L46
  constraint vertical L47
extrude "Extrude22" cut sketch "Sketch26" against normal blind 30 contours L44 L45 L46 L47
sketch "Sketch27" plane through (0, 30, 0) normal (0, 1, 0) x (-1, 0, 0)
  line L0 (-84, 49) -> (-84, 69)
  line L1 (-84, 69) -> (-59, 69)
  line L2 (-59, 69) -> (-59, 49)
  line L3 (-59, 49) -> (-84, 49)
  line L4 (-57, 49) -> (-57, 69)
  line L5 (-57, 69) -> (-32, 69)
  line L6 (-32, 69) -> (-32, 49)
  line L7 (-32, 49) -> (-57, 49)
  line L8 (-30, 49) -> (-30, 69)
  line L9 (-30, 69) -> (-5, 69)
  line L10 (-5, 69) -> (-5, 49)
  line L11 (-5, 49) -> (-30, 49)
  line L12 (-111, 27) -> (-111, 47)
  line L13 (-111, 47) -> (-86, 47)
  line L14 (-86, 47) -> (-86, 27)
  line L15 (-86, 27) -> (-111, 27)
  line L16 (-84, 27) -> (-84, 47)
  line L17 (-84, 47) -> (-59, 47)
  line L18 (-59, 47) -> (-59, 27)
  line L19 (-59, 27) -> (-84, 27)
  line L20 (-57, 27) -> (-57, 47)
  line L21 (-57, 47) -> (-32, 47)
  line L22 (-32, 47) -> (-32, 27)
  line L23 (-32, 27) -> (-57, 27)
  line L24 (-30, 27) -> (-30, 47)
  line L25 (-30, 47) -> (-5, 47)
  line L26 (-5, 47) -> (-5, 27)
  line L27 (-5, 27) -> (-30, 27)
  line L28 (-111, 25) -> (-86, 25)
  line L29 (-86, 25) -> (-86, 5)
  line L30 (-86, 5) -> (-111, 5)
  line L31 (-111, 5) -> (-111, 25)
  line L32 (-84, 5) -> (-84, 25)
  line L33 (-84, 25) -> (-59, 25)
  line L34 (-59, 25) -> (-59, 5)
  line L35 (-59, 5) -> (-84, 5)
  line L36 (-57, 5) -> (-57, 25)
  line L37 (-57, 25) -> (-32, 25)
  line L38 (-32, 25) -> (-32, 5)
  line L39 (-32, 5) -> (-57, 5)
  line L40 (-30, 5) -> (-30, 25)
  line L41 (-30, 25) -> (-5, 25)
  line L42 (-5, 25) -> (-5, 5)
  line L43 (-5, 5) -> (-30, 5)
  line L44 (-116, 98) -> (-116, 0)
  line L45 (-116, 0) -> (0, 0)
  line L46 (0, 0) -> (0, 98)
  line L47 (0, 98) -> (-116, 98)
  line L48 (-86, 49) -> (-111, 49)
  line L49 (-111, 49) -> (-111, 69)
  line L50 (-111, 69) -> (-86, 69)
  line L51 (-86, 69) -> (-86, 49)
  constraint horizontal L48
  constraint vertical L49
  constraint horizontal L50
  constraint vertical L51
extrude "Extrude23" cut sketch "Sketch27" against normal blind 30 contours L48 L49 L50 L51
sketch "Sketch28" plane through (0, 30, 0) normal (0, 1, 0) x (-1, 0, 0)
  line L0 (-111, 49) -> (-111, 69)
  line L1 (-111, 69) -> (-86, 69)
  line L2 (-86, 69) -> (-86, 49)
  line L3 (-86, 49) -> (-111, 49)
  line L4 (-84, 49) -> (-84, 69)
  line L5 (-84, 69) -> (-59, 69)
  line L6 (-59, 69) -> (-59, 49)
  line L7 (-59, 49) -> (-84, 49)
  line L8 (-57, 49) -> (-57, 69)
  line L9 (-57, 69) -> (-32, 69)
  line L10 (-32, 69) -> (-32, 49)
  line L11 (-32, 49) -> (-57, 49)
  line L12 (-30, 49) -> (-30, 69)
  line L13 (-30, 69) -> (-5, 69)
  line L14 (-5, 69) -> (-5, 49)
  line L15 (-5, 49) -> (-30, 49)
  line L16 (-111, 27) -> (-111, 47)
  line L17 (-111, 47) -> (-86, 47)
  line L18 (-86, 47) -> (-86, 27)
  line L19 (-86, 27) -> (-111, 27)
  line L20 (-84, 27) -> (-84, 47)
  line L21 (-84, 47) -> (-59, 47)
  line L22 (-59, 47) -> (-59, 27)
  line L23 (-59, 27) -> (-84, 27)
  line L24 (-57, 27) -> (-57, 47)
  line L25 (-57, 47) -> (-32, 47)
  line L26 (-32, 47) -> (-32, 27)
  line L27 (-32, 27) -> (-57, 27)
  line L28 (-30, 27) -> (-30, 47)
  line L29 (-30, 47) -> (-5, 47)
  line L30 (-5, 47) -> (-5, 27)
  line L31 (-5, 27) -> (-30, 27)
  line L32 (-111, 25) -> (-86, 25)
  line L33 (-86, 25) -> (-86, 5)
  line L34 (-86, 5) -> (-111, 5)
  line L35 (-111, 5) -> (-111, 25)
  line L36 (-84, 5) -> (-84, 25)
  line L37 (-84, 25) -> (-59, 25)
  line L38 (-59, 25) -> (-59, 5)
  line L39 (-59, 5) -> (-84, 5)
  line L40 (-57, 5) -> (-57, 25)
  line L41 (-57, 25) -> (-32, 25)
  line L42 (-32, 25) -> (-32, 5)
  line L43 (-32, 5) -> (-57, 5)
  line L44 (-30, 5) -> (-30, 25)
  line L45 (-30, 25) -> (-5, 25)
  line L46 (-5, 25) -> (-5, 5)
  line L47 (-5, 5) -> (-30, 5)
  line L48 (-116, 98) -> (-116, 0)
  line L49 (-116, 0) -> (0, 0)
  line L50 (0, 0) -> (0, 98)
  line L51 (0, 98) -> (-116, 98)
  line L52 (-5, 71) -> (-30, 71)
  line L53 (-30, 71) -> (-30, 91)
  line L54 (-30, 91) -> (-5, 91)
  line L55 (-5, 91) -> (-5, 71)
  constraint horizontal L52
  constraint vertical L53
  constraint horizontal L54
  constraint vertical L55
extrude "Extrude24" cut sketch "Sketch28" against normal blind 30 contours L52 L53 L54 L55
sketch "Sketch29" plane through (0, 30, 0) normal (0, 1, 0) x (-1, 0, 0)
  line L0 (-30, 71) -> (-30, 91)
  line L1 (-30, 91) -> (-5, 91)
  line L2 (-5, 91) -> (-5, 71)
  line L3 (-5, 71) -> (-30, 71)
  line L4 (-111, 49) -> (-111, 69)
  line L5 (-111, 69) -> (-86, 69)
  line L6 (-86, 69) -> (-86, 49)
  line L7 (-86, 49) -> (-111, 49)
  line L8 (-84, 49) -> (-84, 69)
  line L9 (-84, 69) -> (-59, 69)
  line L10 (-59, 69) -> (-59, 49)
  line L11 (-59, 49) -> (-84, 49)
  line L12 (-57, 49) -> (-57, 69)
  line L13 (-57, 69) -> (-32, 69)
  line L14 (-32, 69) -> (-32, 49)
  line L15 (-32, 49) -> (-57, 49)
  line L16 (-30, 49) -> (-30, 69)
  line L17 (-30, 69) -> (-5, 69)
  line L18 (-5, 69) -> (-5, 49)
  line L19 (-5, 49) -> (-30, 49)
  line L20 (-111, 27) -> (-111, 47)
  line L21 (-111, 47) -> (-86, 47)
  line L22 (-86, 47) -> (-86, 27)
  line L23 (-86, 27) -> (-111, 27)
  line L24 (-84, 27) -> (-84, 47)
  line L25 (-84, 47) -> (-59, 47)
  line L26 (-59, 47) -> (-59, 27)
  line L27 (-59, 27) -> (-84, 27)
  line L28 (-57, 27) -> (-57, 47)
  line L29 (-57, 47) -> (-32, 47)
  line L30 (-32, 47) -> (-32, 27)
  line L31 (-32, 27) -> (-57, 27)
  line L32 (-30, 27) -> (-30, 47)
  line L33 (-30, 47) -> (-5, 47)
  line L34 (-5, 47) -> (-5, 27)
  line L35 (-5, 27) -> (-30, 27)
  line L36 (-111, 25) -> (-86, 25)
  line L37 (-86, 25) -> (-86, 5)
  line L38 (-86, 5) -> (-111, 5)
  line L39 (-111, 5) -> (-111, 25)
  line L40 (-84, 5) -> (-84, 25)
  line L41 (-84, 25) -> (-59, 25)
  line L42 (-59, 25) -> (-59, 5)
  line L43 (-59, 5) -> (-84, 5)
  line L44 (-57, 5) -> (-57, 25)
  line L45 (-57, 25) -> (-32, 25)
  line L46 (-32, 25) -> (-32, 5)
  line L47 (-32, 5) -> (-57, 5)
  line L48 (-30, 5) -> (-30, 25)
  line L49 (-30, 25) -> (-5, 25)
  line L50 (-5, 25) -> (-5, 5)
  line L51 (-5, 5) -> (-30, 5)
  line L52 (-116, 98) -> (-116, 0)
  line L53 (-116, 0) -> (0, 0)
  line L54 (0, 0) -> (0, 98)
  line L55 (0, 98) -> (-116, 98)
  line L56 (-32, 71) -> (-57, 71)
  line L57 (-57, 71) -> (-57, 91)
  line L58 (-57, 91) -> (-32, 91)
  line L59 (-32, 91) -> (-32, 71)
  constraint horizontal L56
  constraint vertical L57
  constraint horizontal L58
  constraint vertical L59
extrude "Extrude25" cut sketch "Sketch29" against normal blind 30 contours L56 L57 L58 L59
sketch "Sketch30" plane through (0, 30, 0) normal (0, 1, 0) x (-1, 0, 0)
  line L0 (-57, 71) -> (-57, 91)
  line L1 (-57, 91) -> (-32, 91)
  line L2 (-32, 91) -> (-32, 71)
  line L3 (-32, 71) -> (-57, 71)
  line L4 (-30, 71) -> (-30, 91)
  line L5 (-30, 91) -> (-5, 91)
  line L6 (-5, 91) -> (-5, 71)
  line L7 (-5, 71) -> (-30, 71)
  line L8 (-111, 49) -> (-111, 69)
  line L9 (-111, 69) -> (-86, 69)
  line L10 (-86, 69) -> (-86, 49)
  line L11 (-86, 49) -> (-111, 49)
  line L12 (-84, 49) -> (-84, 69)
  line L13 (-84, 69) -> (-59, 69)
  line L14 (-59, 69) -> (-59, 49)
  line L15 (-59, 49) -> (-84, 49)
  line L16 (-57, 49) -> (-57, 69)
  line L17 (-57, 69) -> (-32, 69)
  line L18 (-32, 69) -> (-32, 49)
  line L19 (-32, 49) -> (-57, 49)
  line L20 (-30, 49) -> (-30, 69)
  line L21 (-30, 69) -> (-5, 69)
  line L22 (-5, 69) -> (-5, 49)
  line L23 (-5, 49) -> (-30, 49)
  line L24 (-111, 27) -> (-111, 47)
  line L25 (-111, 47) -> (-86, 47)
  line L26 (-86, 47) -> (-86, 27)
  line L27 (-86, 27) -> (-111, 27)
  line L28 (-84, 27) -> (-84, 47)
  line L29 (-84, 47) -> (-59, 47)
  line L30 (-59, 47) -> (-59, 27)
  line L31 (-59, 27) -> (-84, 27)
  line L32 (-57, 27) -> (-57, 47)
  line L33 (-57, 47) -> (-32, 47)
  line L34 (-32, 47) -> (-32, 27)
  line L35 (-32, 27) -> (-57, 27)
  line L36 (-30, 27) -> (-30, 47)
  line L37 (-30, 47) -> (-5, 47)
  line L38 (-5, 47) -> (-5, 27)
  line L39 (-5, 27) -> (-30, 27)
  line L40 (-111, 25) -> (-86, 25)
  line L41 (-86, 25) -> (-86, 5)
  line L42 (-86, 5) -> (-111, 5)
  line L43 (-111, 5) -> (-111, 25)
  line L44 (-84, 5) -> (-84, 25)
  line L45 (-84, 25) -> (-59, 25)
  line L46 (-59, 25) -> (-59, 5)
  line L47 (-59, 5) -> (-84, 5)
  line L48 (-57, 5) -> (-57, 25)
  line L49 (-57, 25) -> (-32, 25)
  line L50 (-32, 25) -> (-32, 5)
  line L51 (-32, 5) -> (-57, 5)
  line L52 (-30, 5) -> (-30, 25)
  line L53 (-30, 25) -> (-5, 25)
  line L54 (-5, 25) -> (-5, 5)
  line L55 (-5, 5) -> (-30, 5)
  line L56 (-116, 98) -> (-116, 0)
  line L57 (-116, 0) -> (0, 0)
  line L58 (0, 0) -> (0, 98)
  line L59 (0, 98) -> (-116, 98)
  line L60 (-59, 71) -> (-84, 71)
  line L61 (-84, 71) -> (-84, 91)
  line L62 (-84, 91) -> (-59, 91)
  line L63 (-59, 91) -> (-59, 71)
  constraint horizontal L60
  constraint vertical L61
  constraint horizontal L62
  constraint vertical L63
extrude "Extrude26" cut sketch "Sketch30" against normal blind 30 contours L60 L61 L62 L63
sketch "Sketch31" plane through (0, 30, 0) normal (0, 1, 0) x (-1, 0, 0)
  line L0 (-84, 71) -> (-84, 91)
  line L1 (-84, 91) -> (-59, 91)
  line L2 (-59, 91) -> (-59, 71)
  line L3 (-59, 71) -> (-84, 71)
  line L4 (-57, 71) -> (-57, 91)
  line L5 (-57, 91) -> (-32, 91)
  line L6 (-32, 91) -> (-32, 71)
  line L7 (-32, 71) -> (-57, 71)
  line L8 (-30, 71) -> (-30, 91)
  line L9 (-30, 91) -> (-5, 91)
  line L10 (-5, 91) -> (-5, 71)
  line L11 (-5, 71) -> (-30, 71)
  line L12 (-111, 49) -> (-111, 69)
  line L13 (-111, 69) -> (-86, 69)
  line L14 (-86, 69) -> (-86, 49)
  line L15 (-86, 49) -> (-111, 49)
  line L16 (-84, 49) -> (-84, 69)
  line L17 (-84, 69) -> (-59, 69)
  line L18 (-59, 69) -> (-59, 49)
  line L19 (-59, 49) -> (-84, 49)
  line L20 (-57, 49) -> (-57, 69)
  line L21 (-57, 69) -> (-32, 69)
  line L22 (-32, 69) -> (-32, 49)
  line L23 (-32, 49) -> (-57, 49)
  line L24 (-30, 49) -> (-30, 69)
  line L25 (-30, 69) -> (-5, 69)
  line L26 (-5, 69) -> (-5, 49)
  line L27 (-5, 49) -> (-30, 49)
  line L28 (-111, 27) -> (-111, 47)
  line L29 (-111, 47) -> (-86, 47)
  line L30 (-86, 47) -> (-86, 27)
  line L31 (-86, 27) -> (-111, 27)
  line L32 (-84, 27) -> (-84, 47)
  line L33 (-84, 47) -> (-59, 47)
  line L34 (-59, 47) -> (-59, 27)
  line L35 (-59, 27) -> (-84, 27)
  line L36 (-57, 27) -> (-57, 47)
  line L37 (-57, 47) -> (-32, 47)
  line L38 (-32, 47) -> (-32, 27)
  line L39 (-32, 27) -> (-57, 27)
  line L40 (-30, 27) -> (-30, 47)
  line L41 (-30, 47) -> (-5, 47)
  line L42 (-5, 47) -> (-5, 27)
  line L43 (-5, 27) -> (-30, 27)
  line L44 (-111, 25) -> (-86, 25)
  line L45 (-86, 25) -> (-86, 5)
  line L46 (-86, 5) -> (-111, 5)
  line L47 (-111, 5) -> (-111, 25)
  line L48 (-84, 5) -> (-84, 25)
  line L49 (-84, 25) -> (-59, 25)
  line L50 (-59, 25) -> (-59, 5)
  line L51 (-59, 5) -> (-84, 5)
  line L52 (-57, 5) -> (-57, 25)
  line L53 (-57, 25) -> (-32, 25)
  line L54 (-32, 25) -> (-32, 5)
  line L55 (-32, 5) -> (-57, 5)
  line L56 (-30, 5) -> (-30, 25)
  line L57 (-30, 25) -> (-5, 25)
  line L58 (-5, 25) -> (-5, 5)
  line L59 (-5, 5) -> (-30, 5)
  line L60 (-116, 98) -> (-116, 0)
  line L61 (-116, 0) -> (0, 0)
  line L62 (0, 0) -> (0, 98)
  line L63 (0, 98) -> (-116, 98)
  line L64 (-86, 71) -> (-111, 71)
  line L65 (-111, 71) -> (-111, 91)
  line L66 (-111, 91) -> (-86, 91)
  line L67 (-86, 91) -> (-86, 71)
  constraint horizontal L64
  constraint vertical L65
  constraint horizontal L66
  constraint vertical L67
extrude "Extrude27" cut sketch "Sketch31" against normal blind 30 contours L64 L65 L66 L67
sketch "Sketch32" plane through (0, 0, 98) normal (0, 0, 1) x (1, 0, 0)
  line L0 (116, 30) -> (0, 30)
  line L1 (0, 30) -> (0, 0)
  line L2 (0, 0) -> (116, 0)
  line L3 (116, 0) -> (116, 30)
  line L4 (0, 30) -> (10, 30)
  line L5 (10, 30) -> (12, 30)
  line L6 (12, 30) -> (12, 0)
  line L7 (12, 0) -> (10, 0)
  line L8 (10, 0) -> (10, 30)
  constraint coincident L0.end L1.start
  constraint coincident L0 L4.end
  constraint perpendicular L1 L4
  constraint horizontal L5
  constraint vertical L6
  constraint horizontal L7
  constraint vertical L8
  constraint coincident L2 L6.end
extrude "Extrude28" cut sketch "Sketch32" against normal blind 3 contours L0 L2 L5 L6 L7 L8
sketch "Sketch33" plane through (0, 0, 98) normal (0, 0, 1) x (1, 0, 0)
  line L0 (12, 30) -> (12, 0)
  line L1 (12, 0) -> (116, 0)
  line L2 (116, 0) -> (116, 30)
  line L3 (116, 30) -> (12, 30)
  line L4 (116, 30) -> (106, 30)
  line L5 (106, 30) -> (104, 30)
  line L6 (104, 30) -> (104, 0)
  line L7 (104, 0) -> (106, 0)
  line L8 (106, 0) -> (106, 30)
  constraint coincident L2.end L3.start
  constraint coincident L3 L4.end
  constraint perpendicular L2 L4
  constraint horizontal L5
  constraint vertical L6
  constraint horizontal L7
  constraint vertical L8
  constraint coincident L1 L6.end
extrude "Extrude29" cut sketch "Sketch33" against normal blind 3 contours L1 L3 L5 L6 L7 L8
sketch "Sketch34" plane through (0, 0, 95) normal (0, 0, 1) x (1, 0, 0)
  line L0 (10, 0) -> (12, 0)
  line L1 (12, 0) -> (12, 30)
  line L2 (12, 30) -> (10, 30)
  line L3 (10, 30) -> (10, 0)
sketch "Sketch35" plane through (0, 30, 0) normal (0, 1, 0) x (-1, 0, 0)
  line L0 (-106, 95) -> (-106, 98)
  line L1 (-106, 98) -> (-116, 98)
  line L2 (-116, 98) -> (-116, 0)
  line L3 (-116, 0) -> (0, 0)
  line L4 (0, 0) -> (0, 98)
  line L5 (0, 98) -> (-10, 98)
  line L6 (-10, 98) -> (-10, 95)
  line L7 (-10, 95) -> (-12, 95)
  line L8 (-12, 95) -> (-12, 98)
  line L9 (-12, 98) -> (-104, 98)
  line L10 (-104, 98) -> (-104, 95)
  line L11 (-104, 95) -> (-106, 95)
  line L12 (-30, 5) -> (-30, 25)
  line L13 (-30, 25) -> (-5, 25)
  line L14 (-5, 25) -> (-5, 5)
  line L15 (-5, 5) -> (-30, 5)
  line L16 (-57, 5) -> (-57, 25)
  line L17 (-57, 25) -> (-32, 25)
  line L18 (-32, 25) -> (-32, 5)
  line L19 (-32, 5) -> (-57, 5)
  line L20 (-84, 5) -> (-84, 25)
  line L21 (-84, 25) -> (-59, 25)
  line L22 (-59, 25) -> (-59, 5)
  line L23 (-59, 5) -> (-84, 5)
  line L24 (-111, 25) -> (-86, 25)
  line L25 (-86, 25) -> (-86, 5)
  line L26 (-86, 5) -> (-111, 5)
  line L27 (-111, 5) -> (-111, 25)
  line L28 (-30, 27) -> (-30, 47)
  line L29 (-30, 47) -> (-5, 47)
  line L30 (-5, 47) -> (-5, 27)
  line L31 (-5, 27) -> (-30, 27)
  line L32 (-57, 27) -> (-57, 47)
  line L33 (-57, 47) -> (-32, 47)
  line L34 (-32, 47) -> (-32, 27)
  line L35 (-32, 27) -> (-57, 27)
  line L36 (-84, 27) -> (-84, 47)
  line L37 (-84, 47) -> (-59, 47)
  line L38 (-59, 47) -> (-59, 27)
  line L39 (-59, 27) -> (-84, 27)
  line L40 (-111, 27) -> (-111, 47)
  line L41 (-111, 47) -> (-86, 47)
  line L42 (-86, 47) -> (-86, 27)
  line L43 (-86, 27) -> (-111, 27)
  line L44 (-30, 49) -> (-30, 69)
  line L45 (-30, 69) -> (-5, 69)
  line L46 (-5, 69) -> (-5, 49)
  line L47 (-5, 49) -> (-30, 49)
  line L48 (-57, 49) -> (-57, 69)
  line L49 (-57, 69) -> (-32, 69)
  line L50 (-32, 69) -> (-32, 49)
  line L51 (-32, 49) -> (-57, 49)
  line L52 (-84, 49) -> (-84, 69)
  line L53 (-84, 69) -> (-59, 69)
  line L54 (-59, 69) -> (-59, 49)
  line L55 (-59, 49) -> (-84, 49)
  line L56 (-111, 49) -> (-111, 69)
  line L57 (-111, 69) -> (-86, 69)
  line L58 (-86, 69) -> (-86, 49)
  line L59 (-86, 49) -> (-111, 49)
  line L60 (-30, 71) -> (-30, 91)
  line L61 (-30, 91) -> (-5, 91)
  line L62 (-5, 91) -> (-5, 71)
  line L63 (-5, 71) -> (-30, 71)
  line L64 (-57, 71) -> (-57, 91)
  line L65 (-57, 91) -> (-32, 91)
  line L66 (-32, 91) -> (-32, 71)
  line L67 (-32, 71) -> (-57, 71)
  line L68 (-84, 71) -> (-84, 91)
  line L69 (-84, 91) -> (-59, 91)
  line L70 (-59, 91) -> (-59, 71)
  line L71 (-59, 71) -> (-84, 71)
  line L72 (-111, 71) -> (-111, 91)
  line L73 (-111, 91) -> (-86, 91)
  line L74 (-86, 91) -> (-86, 71)
  line L75 (-86, 71) -> (-111, 71)
